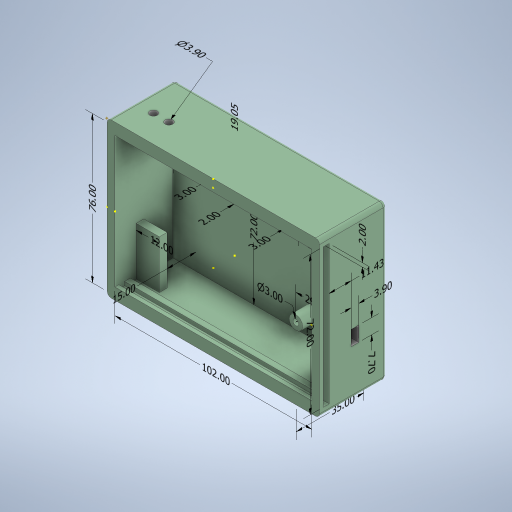
# Autodesk Inventor part: BoxV2
Saved by Autodesk Inventor 2024 (Build 280153000, 153)
## iProperties
Created: 2023-10-23
Part Number: BoxV2
Material: Generic
Document SubType Name: Modeling
Designer: zuhan
Density: 1 g/cm^3
Appearance: Default
Author: zuhan
Autodesk Inventor part; units mm, degrees
ref_plane "YZ Plane" through (0, 0, 0) normal (1, 0, 0) x (0, 1, 0)
ref_plane "XZ Plane" through (0, 0, 0) normal (0, 1, 0) x (-1, 0, 0)
ref_plane "XY Plane" through (0, 0, 0) normal (0, 0, 1) x (1, 0, 0)
sketch "Sketch1" plane through (0, 0, 0) normal (0, 0, 1) x (1, 0, 0)
  point P0 (0, 0)
sketch "Sketch2" plane through (0, 0, 0) normal (0, 0, 1) x (1, 0, 0)
  point P0 (0, 0)
sketch "Sketch3" plane through (0, 0, 0) normal (0, 0, 1) x (1, 0, 0)
  line L0 (-51, -36) -> (51, -36)
  line L1 (51, -36) -> (51, 36)
  line L2 (51, 36) -> (-51, 36)
  line L3 (-51, 36) -> (-51, -36)
  line L4 (-51, -36) -> (51, 36) construction
  line L5 (51, -36) -> (-51, 36) construction
  line L6 (-55, 40) -> (55, 40)
  line L7 (55, 40) -> (55, -40)
  line L8 (55, -40) -> (-55, -40)
  line L9 (-55, -40) -> (-55, 40)
  line L10 (-55, 40) -> (55, -40) construction
  line L11 (55, 40) -> (-55, -40) construction
  point P0 (0, 0)
  dimension "d0" = 102
  dimension "d1" = 72
  dimension "d2" = 110
  dimension "d3" = 80
  constraints: 24 end point, 4 midpoint, 4 parallel, 2 horizontal, 2 perpendicular
  measures "d0" distance of L0.start L0.end
  measures "d1" distance of L1.end L0.end
  measures "d2" distance of L6.start L6.end
  measures "d3" distance of L6.end L7.end
extrude "Extrusion1" add sketch "Sketch3" against normal blind 35
sketch "Sketch4" plane through (51, -36, 0) normal (-1, 0, 0) x (0, 0, 1)
  point P0 (0, 36)
sketch "Sketch5" plane through (-55, -40, 0) normal (-1, 0, 0) x (0, 0, 1)
  line L0 (0, 80) -> (-35, 80) projected
  line L1 (0, 0) -> (-35, 0) projected
  line L2 (-35, 80) -> (-30, 80)
  line L3 (-30, 80) -> (-30, 0)
  line L4 (-30, 0) -> (-35, 0)
  line L5 (-35, 0) -> (-35, 80)
  point P0 (0, 40)
  point P1 (-30, 80)
  dimension "d6" = 5
  constraints: 8 end point, 2 parallel, 1 horizontal, 1 perpendicular, 1 point on line
  measures "d6" distance of L3.end L4.end
extrude "Extrusion2" add sketch "Sketch5" against normal blind 110
fillet "Fillet1" radius 2 8 edges at (-55, 40, -17.5) (0, 40, -35) (55, 40, -17.5) (-55, 0, -35) (-55, -40, -17.5) (0, -40, -35) (55, 0, -35) (55, -40, -17.5)
sketch "Sketch6" plane through (55, -38, 0) normal (1, 0, 0) x (0, 0, -1)
  line L0 (3, 2) -> (7, 2)
  line L1 (7, 2) -> (7, 74)
  line L2 (7, 74) -> (3, 74)
  line L3 (3, 74) -> (3, 2)
  line L4 (3, 2) -> (7, 74) construction
  line L5 (7, 2) -> (3, 74) construction
  line L6 (0, 0) -> (0, 76) projected
  line L7 (33, 0) -> (0, 0) projected
  point P0 (0, 38)
  point P1 (5, 38)
  point P2 (5, 74)
  dimension "d26" = 3
  dimension "d27" = 2
  dimension "d28" = 72
  dimension "d29" = 4
  constraints: 12 end point, 3 midpoint, 2 parallel, 1 horizontal, 1 perpendicular
  measures "d26" distance between parallel lines of L3 L6
  measures "d27" distance between parallel lines of L7 L0
  measures "d28" distance from line of point (5, 74) L0
  measures "d29" distance between parallel lines of L3 L1
extrude "Extrusion3" cut sketch "Sketch6" against normal blind 10
sketch "Sketch7" plane through (-51, 36, 0) normal (0, -1, 0) x (1, 0, 0)
  point P0 (51, 0)
sketch "Sketch11" plane through (-51, 36, -30) normal (0, 0, 1) x (1, 0, 0)
  circle A0 centre (2.54, -2.54) radius 1.27
  line L0 (0, 0) -> (102, 0) projected
  line L1 (0, -72) -> (0, 0) projected
  circle A1 centre (2.54, -21.59) radius 1.27
  point P0 (51, -36)
  dimension "d44" = 2.54
  dimension "d45" = 2.54
  dimension "d46" = 2.54
  dimension "d47" = 2.54
  dimension "d48" = 2.54
  dimension "d49" = 19.05
  constraints: 2 centre point
  measures "d44" diameter of A0
  measures "d45" distance from line of L0 A0.centre
  measures "d46" distance from line of L1 A0.centre
  measures "d47" diameter of A1
  measures "d48" distance from line of L1 A1.centre
  measures "d49" distance of A0.centre A1.centre
extrude "Extrusion6" add sketch "Sketch11" along normal blind 2
sketch "Sketch12" plane through (-55, -38, 0) normal (-1, 0, 0) x (0, 0, 1)
  point P0 (0, 38)
sketch "Sketch13" plane through (-55, -38, 0) normal (-1, 0, 0) x (0, 0, 1)
  line L0 (0, 76) -> (0, 0) projected
  line L1 (0, 76) -> (-8, 76)
  line L2 (-8, 76) -> (-8, 0)
  line L3 (-8, 0) -> (0, 0)
  line L4 (0, 0) -> (0, 76)
  point P0 (0, 38)
  point P1 (-4, 0)
  point P2 (-4, 76)
  dimension "d52" = 8
  dimension "d53" = 76
  constraints: 8 end point, 2 midpoint, 2 parallel, 1 horizontal, 1 perpendicular
  measures "d52" distance of L3.end L2.end
  measures "d53" distance of point (-4, 0) point (-4, 76)
extrude "Extrusion7" add sketch "Sketch13" against normal blind 110
sketch "Sketch14" plane through (55, -38, 0) normal (1, 0, 0) x (0, 0, -1)
  line L0 (2, 2) -> (5, 2)
  line L1 (5, 2) -> (5, 74)
  line L2 (5, 74) -> (2, 74)
  line L3 (2, 74) -> (2, 2)
  line L4 (0, 0) -> (0, 76) projected
  line L5 (33, 0) -> (0, 0) projected
  point P0 (0, 38)
  point P1 (3.5, 2)
  dimension "d56" = 3
  dimension "d57" = 2
  dimension "d58" = 72
  dimension "d59" = 2
  constraints: 8 end point, 2 parallel, 1 horizontal, 1 midpoint, 1 perpendicular
  measures "d56" distance between parallel lines of L1 L3
  measures "d57" distance between parallel lines of L4 L3
  measures "d58" distance of L0.end L1.end
  measures "d59" distance from line of L5 point (3.5, 2)
extrude "Extrusion8" cut sketch "Sketch14" against normal blind 106
sketch "Sketch15" plane through (0, 0, 0) normal (0, 0, 1) x (1, 0, 0)
  line L0 (-51, 34) -> (51, 34)
  line L1 (51, 34) -> (51, -34)
  line L2 (51, -34) -> (-51, -34)
  line L3 (-51, -34) -> (-51, 34)
  line L4 (-51, 34) -> (51, -34) construction
  line L5 (51, 34) -> (-51, -34) construction
  point P0 (0, 0)
  dimension "d62" = 102
  dimension "d63" = 68
  constraints: 12 end point, 2 midpoint, 2 parallel, 1 horizontal, 1 perpendicular
  measures "d62" distance of L1.end L2.end
  measures "d63" distance of L0.end L1.end
extrude "Extrusion9" cut sketch "Sketch15" against normal blind 10
sketch "Sketch16" plane through (-51, -36, -30) normal (1, 0, 0) x (0, 0, -1)
  point P0 (-30, 36)
sketch "Sketch17" plane through (-55, -38, 0) normal (-1, 0, 0) x (0, 0, 1)
  line L0 (-11, 27) -> (-15, 27)
  line L1 (-15, 27) -> (-15, 2)
  line L2 (-15, 2) -> (-11, 2)
  line L3 (-11, 2) -> (-11, 27)
  line L4 (0, 76) -> (0, 0) projected
  line L5 (0, 0) -> (-33, 0) projected
  point P0 (0, 38)
  point P1 (-13, 2)
  point P2 (-13, 27)
  dimension "d96" = 11
  dimension "d97" = 2
  dimension "d98" = 4
  dimension "d99" = 25
  constraints: 8 end point, 2 midpoint, 2 parallel, 1 horizontal, 1 perpendicular
  measures "d96" distance between parallel lines of L4 L3
  measures "d97" distance from line of L5 point (-13, 2)
  measures "d98" distance between parallel lines of L3 L1
  measures "d99" distance from line of L2 point (-13, 27)
extrude "Extrusion10" add sketch "Sketch17" against normal blind 16
sketch "Sketch18" plane through (-51, -36, -11) normal (0, 0, 1) x (1, 0, 0)
  point P0 (51, 36)
sketch "Sketch19" plane through (-51, 36, -30) normal (0, 0, 1) x (1, 0, 0)
  circle A0 centre (74.07, -11.97) radius 1.5
  line L0 (102, 0) -> (102, -72) projected
  line L1 (0, 0) -> (102, 0) projected
  circle A1 centre (72.8, -60.03) radius 1.5
  line L2 (102, -72) -> (0, -72) projected
  circle A2 centre (74.07, -11.97) radius 3.5
  circle A3 centre (72.8, -60.03) radius 3.5
  point P0 (51, -36)
  dimension "d102" = 3
  dimension "d103" = 27.93
  dimension "d104" = 11.97
  dimension "d105" = 3
  dimension "d106" = 29.2
  dimension "d107" = 11.97
  dimension "d108" = 7
  dimension "d109" = 7
  constraints: 4 centre point, 2 coincident
  measures "d102" diameter of A0
  measures "d103" distance from line of L0 A0.centre
  measures "d104" distance from line of L1 A0.centre
  measures "d105" diameter of A1
  measures "d106" distance from line of L0 A1.centre
  measures "d107" distance from line of L2 A1.centre
  measures "d108" diameter of A2
  measures "d109" diameter of A3
extrude "Extrusion11" add sketch "Sketch19" along normal blind 9.03
sketch "Sketch20" plane through (-53, 40, 0) normal (0, 1, 0) x (1, 0, 0)
  point P0 (53, 0)
sketch "Sketch21" plane through (-53, 40, 0) normal (0, 1, 0) x (1, 0, 0)
  circle A0 centre (16, 14) radius 1.95
  line L0 (106, 0) -> (0, 0) projected
  line L1 (106, 33) -> (106, 0) projected
  circle A1 centre (8, 14) radius 1.95
  point P0 (53, 0)
  dimension "d116" = 3.9
  dimension "d117" = 14
  dimension "d118" = 90
  dimension "d119" = 3.9
  dimension "d120" = 8
  dimension "d121" = 14
  constraints: 2 centre point
  measures "d116" diameter of A0
  measures "d117" distance from line of L0 A0.centre
  measures "d118" distance from line of L1 A0.centre
  measures "d119" diameter of A1
  measures "d120" distance of A0.centre A1.centre
  measures "d121" distance from line of L0 A1.centre
extrude "Extrusion12" cut sketch "Sketch21" against normal blind 10
sketch "Sketch22" plane through (55, -38, 0) normal (1, 0, 0) x (0, 0, -1)
  line L0 (16.43, 21.99) -> (20.33, 21.99)
  line L1 (20.33, 21.99) -> (20.33, 29.69)
  line L2 (20.33, 29.69) -> (16.43, 29.69)
  line L3 (16.43, 29.69) -> (16.43, 21.99)
  line L4 (33, 0) -> (0, 0) projected
  line L5 (5, 74) -> (5, 2) projected
  point P0 (0, 38)
  point P1 (18.38, 21.99)
  point P2 (16.43, 25.84)
  dimension "d140" = 21.99
  dimension "d141" = 3.9
  dimension "d142" = 7.7
  dimension "d143" = 11.43
  constraints: 8 end point, 2 midpoint, 2 parallel, 1 horizontal, 1 perpendicular
  measures "d140" distance from line of L4 point (18.38, 21.99)
  measures "d141" distance between parallel lines of L1 L3
  measures "d142" distance between parallel lines of L0 L2
  measures "d143" distance from line of L5 point (16.43, 25.84)
extrude "Extrusion13" cut sketch "Sketch22" against normal blind 10
sketch "Sketch8" plane through (-53, -40, 0) normal (0, -1, 0) x (1, 0, 0)
  line L0 (2, 0) -> (104, 0)
  line L1 (104, 0) -> (104, -3)
  line L2 (104, -3) -> (2, -3)
  line L3 (2, -3) -> (2, 0)
  line L4 (0, 0) -> (106, 0) projected
  line L5 (0, -33) -> (0, 0) projected
  point P0 (53, 0)
  point P1 (2, -1.5)
  point P2 (104, -1.5)
  dimension "d32" = 0
  dimension "d33" = 3
  dimension "d34" = 2
  dimension "d35" = 102
  constraints: 8 end point, 2 midpoint, 2 parallel, 1 horizontal, 1 perpendicular
  measures "d32" distance between parallel lines of L4 L0
  measures "d33" distance between parallel lines of L0 L2
  measures "d34" distance from line of L5 point (2, -1.5)
  measures "d35" distance of point (2, -1.5) point (104, -1.5)
sketch "Sketch9" plane through (0, 0, 0) normal (0, 0, 1) x (1, 0, 0)
  line L0 (-51, 35) -> (51, 35)
  line L1 (51, 35) -> (51, -35)
  line L2 (51, -35) -> (-51, -35)
  line L3 (-51, -35) -> (-51, 35)
  line L4 (-51, 35) -> (51, -35) construction
  line L5 (51, 35) -> (-51, -35) construction
  point P0 (0, 0)
  dimension "d39" = 102
  dimension "d40" = 70
  constraints: 12 end point, 2 midpoint, 2 parallel, 1 horizontal, 1 perpendicular
  measures "d39" distance of L1.end L2.end
  measures "d40" distance between parallel lines of L0 L2
body "Solid1"
